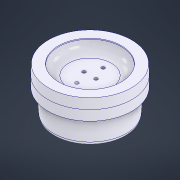
# Autodesk Inventor part: 020
Saved by Autodesk Inventor 2022 (Build 260153000, 153)
## iProperties
Created: 2021-11-03
Part Number: 020
Material: Concrete
Document SubType Name: Modeling
Designer: vinicius.miguel
Density: 2.40731 g/cm^3
Appearance: Cool White
Mass: 367.791 g
Surface Area: 249.915 cm^2
Volume: 152.781 cm^3
Author: vinicius.miguel
Autodesk Inventor part; units mm, degrees
ref_plane "YZ Plane" through (0, 0, 0) normal (1, 0, 0) x (0, 1, 0)
ref_plane "XZ Plane" through (0, 0, 0) normal (0, 1, 0) x (-1, 0, 0)
sketch "Sketch1" plane through (0, 0, 0) normal (0, 0, 1) x (1, 0, 0)
  arc A0 (-35.9893, 3.2169) -> (-30.1047, 1.1907) centre (-32.6581, 3.3332) ccw
  line L0 (-30.1047, 1.1907) -> (-16, 18)
  line L1 (-41.5, 35) -> (-41.5, 25)
  line L2 (-41.5, 25) -> (-36.75, 25)
  line L3 (0, 0) -> (0, 35) construction
  line L4 (0, 0) -> (-46.1303, 0) construction
  line L5 (-16, 18) -> (-16, 35)
  line L6 (-16, 35) -> (-41.5, 35)
  line L7 (-16, 18) -> (0, 18)
  line L8 (0, 18) -> (0, 35)
  line L9 (-16, 35) -> (0, 35)
  line L10 (-41.5, 35) -> (-41.1508, 45)
  line L11 (-41.1508, 45) -> (-31.1508, 45)
  line L12 (-31.1508, 45) -> (-30.2759, 35)
  line L13 (-36.75, 25) -> (-35.9893, 3.2169)
  dimension "d0" = 32
  dimension "d2" = 18
  dimension "d4" = 83
  dimension "d20" = 35
  dimension "d21" = 140
  dimension "d22" = 10
  dimension "d44" = 95
  dimension "d45" = 10
  dimension "d46" = 92
  dimension "d48" = 73.5
  dimension "d49" = 92
  dimension "d73" = 45
  constraints: 28 end point, 4 perpendicular, 3 tangent, 2 point on circle, 2 point on line, 1 centre point, 1 collinear, 1 horizontal, 1 horizontal alignment, 1 parallel, 1 vertical
  measures "d0" diameter of L0.end L3
  measures "d2" vertical distance of L0.end L3.start
  measures "d4" diameter of L1 L3
  measures "d20" distance from line of L6 L3.start
  measures "d21" angle of L0 L5
  measures "d22" distance of L1.start L1.end
  measures "d44" angle of L12 L11
  measures "d45" distance of L10.end L11.end
  measures "d46" angle of L10 L11
  measures "d48" diameter of L2.end L3
  measures "d49" angle of L13 L2
  measures "d73" distance from line of L11 L3.start
revolve "Revolution1" add sketch "Sketch1" angle 360 about axis through (0, 0, 0) along (0, 1, 0)
fillet "Fillet1" radius 10 1 edges at (30.2759, 35, 0)
sketch "Sketch3" plane through (0, 18, 0) normal (0, -1, 0) x (1, 0, 0)
  circle A0 centre (-6, 0) radius 1.6
  circle A1 centre (6, 0) radius 1.6
  circle A2 centre (0, 13) radius 1.6
  circle A3 centre (-11.2583, 6.5) radius 1.6
  circle A4 centre (-11.2583, -6.5) radius 1.6
  circle A5 centre (0, -13) radius 1.6
  circle A6 centre (11.2583, -6.5) radius 1.6
  circle A7 centre (11.2583, 6.5) radius 1.6
  point P0 (0, 0)
  dimension "d50" = 3.2
  dimension "d51" = 3.2
  dimension "d52" = 6
  dimension "d53" = 6
  dimension "d54" = 3.2
  dimension "d55" = 13
  dimension "d58" = 360
  constraints: 8 centre point, 2 horizontal alignment, 1 vertical alignment, 13 other
  measures "d50" diameter of A0
  measures "d51" diameter of A1
  measures "d52" distance of point (0, 0) A0.centre
  measures "d53" distance of point (0, 0) A1.centre
  measures "d54" diameter of A2
  measures "d55" distance of A2.centre point (0, 0)
extrude "Extrusion1" cut sketch "Sketch3" against normal through all contours A0 | A1 | A2 | A5
sketch "Sketch4" plane through (0, 18, 0) normal (0, -1, 0) x (1, 0, 0)
  circle A0 centre (0, 0) radius 10
  circle A1 centre (-6, 0) radius 1.6 projected
  circle A2 centre (6, 0) radius 1.6 projected
  point P0 (0, 0)
  dimension "d62" = 20
  constraints: 1 centre point, 1 coincident
  measures "d62" diameter of A0
extrude "Extrusion2" add sketch "Sketch4" along normal blind 5
ref_plane "Work Plane1" through (0, 30, -41.5) normal (0, 0, 1) x (1, 0, 0)
equation "\"d51\" = d50"
body "Solid1"
